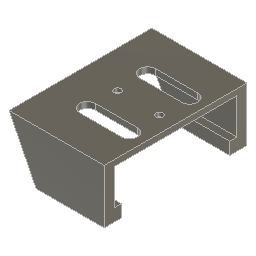
Крепление аккамулятора Makita_ver6 (Autodesk Fusion 360 design; units mm, degrees)
Autodesk Fusion 360 part; units mm, degrees
sketch "Sketch1" plane through (0, 0, 0) normal (0, 0, 1) x (1, 0, 0)
  line L0 (36, 27) -> (-36, 27)
  line L1 (-36, 27) -> (-36, -27)
  line L2 (-36, -27) -> (36, -27)
  line L3 (36, -27) -> (36, 27)
  line L4 (36, 30.6) -> (-36, 30.6)
  line L5 (-36, 35.6) -> (-36, -30.6)
  line L6 (-36, -30.6) -> (36, -30.6)
  line L7 (36, -30.6) -> (36, 30.6)
  line L8 (33, 35.6) -> (-36, 35.6)
  line L9 (41, -27.6) -> (41, 27.6)
  line L10 (33, -35.6) -> (-36, -35.6)
  line L11 (-36, -35.6) -> (-36, 30.6)
  arc A0 (41, 27.6) -> (33, 35.6) centre (33, 27.6) ccw
  arc A1 (33, -35.6) -> (41, -27.6) centre (33, -27.6) ccw
  circle A2 centre (-31, 0) radius 1.75
  line L12 (-31, 11) -> (-10, 11)
  arc A3 (-10, 11) -> (-10, 19) centre (-10, 15) ccw
  line L13 (-10, 19) -> (-31, 19)
  arc A4 (-31, 19) -> (-31, 11) centre (-31, 15) ccw
  line L14 (-31, 15) -> (-10, 15) construction
  line L15 (1.75, 0) -> (22.5, 0)
  line L16 (-31, -11) -> (-10, -11)
  line L17 (-10, -19) -> (-31, -19)
  arc A5 (-10, -19) -> (-10, -11) centre (-10, -15) ccw
  arc A6 (-31, -11) -> (-31, -19) centre (-31, -15) ccw
  circle A7 centre (-10, 0) radius 1.75
  dimension "d1" = 72
  dimension "d2" = 54
  dimension "d3" = 61.2
  dimension "d6" = 8
  dimension "d32" = 3.5
  dimension "d34" = 8
  dimension "d40" = 3.5
  constraint horizontal L0
  constraint perpendicular L0 L1
  constraint parallel L0 L2
  constraint parallel L1 L3
  constraint horizontal L4
  constraint perpendicular L4 L5
  constraint parallel L4 L6
  constraint parallel L5 L7
  constraint coincident L4.end L5
  constraint tangent L9 A0
  constraint tangent L8 A0
  constraint tangent L10 A1
  constraint tangent L9 A1
  constraint equal A0 A1
  constraint tangent L12 A3
  constraint tangent A3 L13
  constraint parallel L12 L13
  constraint tangent L13 A4
  constraint tangent L12 A4
  constraint symmetric L12.start L15 L16.start
  constraint symmetric L12.end L15 L16.end
  constraint symmetric A3.end L15 L17.start
  constraint symmetric L13.end L15 L17.end
  constraint symmetric A3 L15 A5
  constraint symmetric A4 L15 A6
  measures "d1" distance of L1.end L2.end
  measures "d2" distance of L0.end L1.end
  measures "d3" distance of L4.end L5.end
  measures "d6" radius of A0
  measures "d32" diameter of A2
  measures "d34" diameter of A3
  measures "d40" diameter of A7
extrude "Extrude1" add sketch "Sketch1" along normal blind 6.15 contours L3 L4 L5 L6 L7 L8 L9 L10 L11 A0 A1 | L0 L4 L5 L7 L11 | L2 L5 L6 L7 L11
extrude "Extrude2" add sketch "Sketch1" along normal blind 24 contours L3 L4 L5 L6 L7 L8 L9 L10 L11 A0 A1
extrude "Extrude3" add sketch "Sketch1" along normal blind 27 and the other way blind -24
sketch "Sketch2" plane through (0, -35.6, 0) normal (0, -1, 0) x (1, 0, 0)
  line L0 (-36, 0) -> (33, 0)
  line L1 (33, 0) -> (33, 27)
  line L2 (-36, 27) -> (-36, 0)
  line L3 (-36, 0) -> (-49.5029, 27)
  line L4 (-36, 0) -> (-6, 0) construction
  line L5 (-36, 27) -> (-49.5029, 27)
  line L6 (33, 27) -> (-36, 27)
  line L7 (-36, 27) -> (-36, 24)
  line L8 (-36, 24) -> (-36.4845, 24)
  line L9 (-36.4845, 24) -> (-48.0026, 24)
  line L10 (-36, 0) -> (-36, 6.4)
  line L11 (-36, 6.4) -> (-36, 6)
  line L12 (-36, 6.4) -> (-39.2007, 6.4)
  line L13 (-36, 0) -> (-32.4, 0)
  line L14 (-49.5029, 27) -> (-47.5029, 27)
  line L15 (-36, 6.4) -> (-32.4, 6.4)
  line L16 (-32.4, 6.4) -> (-32.4, 0)
  dimension "d11" = 116.57
  dimension "d25" = 6.4
  dimension "d36" = 3.6
  dimension "d37" = 2
  constraint horizontal L4
  constraint coincident L0.start L2.end
  constraint coincident L2.start L5.start
  constraint perpendicular L2 L5
  constraint coincident L2 L7.end
  constraint perpendicular L2 L8
  constraint coincident L3 L9.end
  constraint perpendicular L2 L9
  constraint perpendicular L4 L10
  constraint coincident L2 L11.end
  constraint coincident L3 L12.end
  constraint perpendicular L10 L12
  constraint perpendicular L2 L13
  constraint parallel L5 L14
  constraint perpendicular L11 L15
  measures "d11" angle of L3 L4
  measures "d25" distance of L0.start L10.end
  measures "d36" distance of L0.start L13.end
  measures "d37" distance of L3.end L14.end
extrude "Extrude4" add sketch "Sketch2" against normal blind 5 contours L2 L3 L10 L11 L12 | L2 L3 L8 L9 L12
extrude "Extrude5" add sketch "Sketch2" along normal blind -71.2 and the other way blind 66.2 contours L2 L3 L10 L11 L12 | L2 L3 L8 L9 L12
extrude "Extrude6" add sketch "Sketch2" against normal blind 71.2 contours L2 L3 L5 L7 L8 L9 L14
extrude "Extrude7" cut sketch "Sketch2" along normal blind -8.6 and the other way blind 5 contours L0 L2 L10 L11 L13 L15 L16
extrude "Extrude8" cut sketch "Sketch2" along normal blind -66.2 and the other way blind 62.6 contours L0 L2 L10 L11 L13 L15 L16
chamfer "Chamfer2" distance 1 angle 45 2 edges at (-32.6316, 0.6328, 24) (-11.6316, 0.6328, 24)
sketch "Sketch3" plane through (0, 0, 27) normal (0, 0, 1) x (-1, 0, 0)
  arc A0 (10, 19) -> (10, 11) centre (10, 15) ccw
  line L0 (10, 19) -> (31, 19)
  arc A1 (31, 11) -> (31, 19) centre (31, 15) ccw
  line L1 (31, 11) -> (10, 11)
  circle A2 centre (31, 0) radius 1.75
  circle A3 centre (10, 0) radius 1.75
  arc A4 (31, -19) -> (31, -11) centre (31, -15) ccw
  line L2 (31, -19) -> (10, -19)
  arc A5 (10, -11) -> (10, -19) centre (10, -15) ccw
  line L3 (10, -11) -> (31, -11)
  line L4 (49.5029, 35.6) -> (-33, 35.6)
  arc A6 (-33, 35.6) -> (-41, 27.6) centre (-33, 27.6) ccw
  line L5 (-41, 27.6) -> (-41, -27.6)
  arc A7 (-41, -27.6) -> (-33, -35.6) centre (-33, -27.6) ccw
  line L6 (-33, -35.6) -> (49.5029, -35.6)
  line L7 (49.5029, -35.6) -> (49.5029, 35.6)
  line L8 (2.0837, -40) -> (-45, -40)
  line L9 (-45, -40) -> (-45, 40)
  line L10 (-45, 40) -> (2.0837, 40)
  line L11 (2.0837, 40) -> (2.0837, -40)
  constraint horizontal L8
  constraint vertical L9
  constraint horizontal L10
  constraint vertical L11
extrude "Extrude9" cut sketch "Sketch3" against normal blind 55 contours L4 A6 L5 A7 L6 L11 | L4 A6 L5 A7 L6 L8 L9 L10 L11
chamfer "Chamfer3" distance 1 angle 45 2 edges at (-32.4, -28.8, 6.15) (-32.4, 28.8, 6.15)
